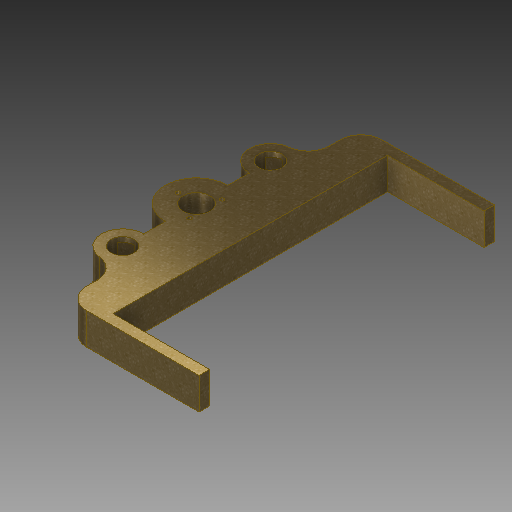
# Autodesk Inventor part: AlteredPlatform
Saved by Autodesk Inventor 2018 (Build 220112000, 112)
## iProperties
Created: 2017-10-12
Part Number: AlteredPlatform
Material: Generic
Document SubType Name: Modeling
Designer: 1452927
Density: 1 g/cm^3
Appearance: Foil Gold
Author: 1452927
Autodesk Inventor part; units mm, degrees
ref_plane "YZ Plane" through (0, 0, 0) normal (1, 0, 0) x (0, 1, 0)
sketch "Sketch1" plane through (0, 0, 0) normal (0, 1, 0) x (-1, 0, 0)
  circle A0 centre (0, 0) radius 8.0645
  circle A1 centre (0, -44.45) radius 6.985
  circle A2 centre (0, 44.45) radius 6.985
  line L0 (-39.6048, 88.9) -> (39.6048, 88.9)
  line L1 (39.6048, 88.9) -> (39.6048, -88.9)
  line L2 (39.6048, -88.9) -> (-39.6048, -88.9)
  line L3 (-39.6048, -88.9) -> (-39.6048, 88.9)
  line L4 (-39.6048, 88.9) -> (39.6048, -88.9) construction
  line L5 (39.6048, 88.9) -> (-39.6048, -88.9) construction
  line L6 (10.9754, 63.5) -> (10.9754, 0) construction
  point P0 (0, 0)
  point P1 (0, 0)
  dimension "d0" = 16.129
  dimension "d1" = 13.97
  dimension "d2" = 13.97
  dimension "d28" = 177.8
  dimension "d82" = 44.45
  dimension "d83" = 44.45
  constraints: 14 end point, 4 midpoint, 3 centre point, 2 coincident, 2 parallel, 1 horizontal, 1 perpendicular, 1 vertical, 4 other
  measures "d0" diameter of A0
  measures "d1" diameter of A1
  measures "d2" diameter of A2
  measures "d28" distance of L0.end L1.end
  measures "d82" distance of A0.centre A1.centre
  measures "d83" distance of point (0, 44.45) A0.centre
extrude "Extrusion4" add sketch "Sketch1" along normal blind 19.05
ref_plane "Work Plane2" through (0, 19.05, 0) normal (0, 1, 0) x (1, 0, 0)
sketch "Sketch2" plane through (0, 19.05, 0) normal (0, 1, 0) x (1, 0, 0)
  circle A0 centre (-11.2395, 0) radius 1.25
  circle A1 centre (0, 0) radius 7.94 projected
  circle A2 centre (5.6197, -9.7337) radius 1.25
  circle A3 centre (5.6198, 9.7337) radius 1.25
  dimension "d11" = 2.5
  dimension "d12" = 11.2395
  dimension "d15" = 360
  constraints: 3 centre point, 7 other
  measures "d11" diameter of A0
  measures "d12" distance of A0.centre A1.centre
ref_plane "Work Plane1" through (0, 19.05, 0) normal (0, 1, 0) x (1, 0, 0)
extrude "Extrusion5" cut sketch "Sketch2" against normal up to next contours A0 | A2 | A3
sketch "Sketch6" plane through (0, 19.05, 0) normal (0, 1, 0) x (1, 0, 0)
  circle A0 centre (0, 0) radius 8.0645 projected
  arc A1 (0, 18.8395) -> (0, -18.8395) centre (0, 0) ccw
  circle A2 centre (-11.2395, 0) radius 1.25 projected
  circle A3 centre (0, -44.45) radius 6.985 projected
  circle A4 centre (0, -44.45) radius 6.985 projected
  arc A5 (0, -31.75) -> (0, -57.15) centre (0, -44.45) ccw
  line L0 (54.9709, 0) -> (-46.1054, 0) construction
  arc A6 (0, 57.15) -> (0, 31.75) centre (0, 44.45) ccw
  line L1 (10.0601, -57.15) -> (10.0601, -88.9)
  line L2 (10.0601, -88.9) -> (-39.6048, -88.9)
  line L3 (-39.6048, 88.9) -> (-39.6048, -88.9) projected
  line L4 (-39.6048, -88.9) -> (-39.6048, 88.9)
  line L5 (-39.6048, 88.9) -> (10.0601, 88.9)
  line L6 (10.0601, 57.15) -> (10.0601, 88.9)
  line L7 (0, 57.15) -> (10.0601, 57.15)
  line L8 (0, 31.75) -> (0, 18.8395)
  line L9 (0, -18.8395) -> (0, -31.75)
  line L10 (10.0601, -57.15) -> (0, -57.15)
  point P0 (0, 0)
  dimension "d77" = 6.35
  dimension "d103" = 12.7
  constraints: 20 end point, 6 point on circle, 4 symmetric about line, 3 centre point, 2 coincident, 2 perpendicular, 2 vertical, 1 collinear, 1 horizontal, 1 tangent, 1 other
  measures "d103" radius of A5
sketch "Sketch12" plane through (0, 19.05, 0) normal (0, 1, 0) x (1, 0, 0)
  line L0 (39.6048, -88.9) -> (39.6048, 88.9) projected
  line L1 (39.6048, -82.55) -> (19.685, -82.55)
  line L2 (19.685, -82.55) -> (19.685, 82.55)
  line L3 (19.685, 82.55) -> (39.6048, 82.55)
  line L4 (39.6048, 82.55) -> (39.6048, -82.55)
  line L5 (39.6048, 88.9) -> (-39.6048, 88.9) projected
  line L6 (-39.6048, -88.9) -> (39.6048, -88.9) projected
  circle A0 centre (0, -44.45) radius 6.985 projected
  point P0 (0, 0)
  point P1 (12.7, 88.9)
  point P2 (12.7, -88.9)
  point P3 (0, 88.9)
  point P4 (10.0601, 88.9)
  point P5 (10.0601, -88.9)
  dimension "d72" = 6.35
  dimension "d73" = 6.35
  dimension "d74" = 12.7
  constraints: 8 end point, 2 parallel, 1 horizontal, 1 perpendicular, 1 point on line
  measures "d72" distance between parallel lines of L5 L3
  measures "d73" distance between parallel lines of L1 L6
  measures "d74" distance edge to line of A0 L2
extrude "Extrusion10" cut sketch "Sketch12" against normal up to next contours L1 L2 L3 L0
sketch "Sketch13" plane through (39.6048, 0, 88.9) normal (1, 0, 0) x (0, 0, -1)
  line L0 (0, 0) -> (0, 19.05) projected
  line L1 (171.45, 0) -> (6.35, 0) projected
  line L2 (0, 19.05) -> (6.35, 19.05)
  line L3 (6.35, 19.05) -> (6.35, 0)
  line L4 (6.35, 0) -> (0, 0)
  line L5 (0, 0) -> (0, 19.05)
  line L6 (171.45, 19.05) -> (171.45, 0) projected
  line L7 (177.8, 19.05) -> (177.8, 0) projected
  line L8 (171.45, 19.05) -> (177.8, 19.05)
  line L9 (177.8, 19.05) -> (177.8, 0)
  line L10 (177.8, 0) -> (171.45, 0)
  line L11 (171.45, 0) -> (171.45, 19.05)
  point P0 (88.9, 0)
  constraints: 16 end point, 4 parallel, 2 horizontal, 2 perpendicular
extrude "Extrusion11" add sketch "Sketch13" along normal blind 50.8
sketch "Sketch14" plane through (19.685, 19.05, 82.55) normal (1, 0, 0) x (0, 0, -1)
  line L0 (0, 0) -> (0, -19.05) projected
  line L1 (165.1, -19.05) -> (0, -19.05) projected
  line L2 (0, 0) -> (165.1, 0)
  line L3 (165.1, 0) -> (165.1, -19.05)
  line L4 (165.1, -19.05) -> (0, -19.05)
  line L5 (0, -19.05) -> (0, 0)
  point P0 (82.55, -19.05)
  constraints: 8 end point, 2 parallel, 1 horizontal, 1 perpendicular
extrude "Extrusion12" add sketch "Sketch14" along normal blind 12.7
extrude "Extrusion14" cut sketch "Sketch6" against normal up to next contours A1 L9 A5 L10 L1 L2 L3 L5 L6 L7 A6 L8
sketch "Sketch16" plane through (0, 19.05, -31.75) normal (-1, 0, 0) x (0, 0, 1)
  line L0 (-15.875, -3.048) -> (-15.875, -16.002)
  line L1 (-19.685, -16.002) -> (-19.685, -3.048)
  line L2 (-19.685, -3.048) -> (-15.875, -3.048)
  line L3 (-9.525, -3.048) -> (-5.715, -3.048)
  line L4 (-19.685, -16.002) -> (-15.875, -16.002)
  line L5 (-9.525, -16.002) -> (-5.715, -16.002)
  line L6 (-5.715, -3.048) -> (-5.715, -16.002)
  line L7 (-9.525, -3.048) -> (-9.525, -16.002)
  point P0 (31.75, -19.05)
  dimension "d106" = 3.81
  dimension "d112" = 3.81
  constraints: 16 end point, 2 horizontal, 1 parallel, 1 perpendicular
  measures "d106" distance between parallel lines of L1 L0
  measures "d112" distance of L3.start L3.end
extrude "Extrusion15" cut sketch "Sketch16" along normal up to next
mirror "Mirror3" about plane through (0, 0, 0) normal (0, 0, 1) of "Extrusion15"
fillet "Fillet8" radius 12.7 4 edges at (10.0601, 9.525, 57.15) (10.0601, 9.525, 88.9) (10.0601, 9.525, -88.9) (10.0601, 9.525, -57.15)
body "Solid2"
